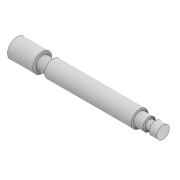
# Autodesk Inventor part: fifth
Saved by Autodesk Inventor 2020 (Build 240168000, 168)
## iProperties
Created: 2021-12-09
Part Number: fifth
Material: Generic
Document SubType Name: Modeling
Designer: NIKHIL VINOD
Density: 1 g/cm^3
Appearance: Default
Author: NIKHIL VINOD
Autodesk Inventor part; units mm, degrees
ref_plane "YZ Plane" through (0, 0, 0) normal (1, 0, 0) x (0, 1, 0)
ref_plane "XZ Plane" through (0, 0, 0) normal (0, 1, 0) x (-1, 0, 0)
ref_plane "XY Plane" through (0, 0, 0) normal (0, 0, 1) x (1, 0, 0)
sketch "Sketch1" plane through (0, 0, 0) normal (0, 0, 1) x (1, 0, 0)
  line L0 (-76.2253, 0) -> (-52.2253, 0)
  line L1 (-52.2253, 6) -> (-52.2253, 9)
  line L2 (-52.2253, 9) -> (-76.2253, 9)
  line L3 (-76.2253, 9) -> (-76.2253, 0)
  line L4 (-52.2253, 0) -> (-42.2253, 0)
  line L5 (-42.2253, 6) -> (-52.2253, 6)
  line L6 (-42.2253, 0) -> (39.7747, 0)
  line L7 (39.7747, 6) -> (39.7747, 8)
  line L8 (39.7747, 8) -> (-42.2253, 8)
  line L9 (-42.2253, 8) -> (-42.2253, 6)
  line L10 (39.7747, 0) -> (48.7747, 0)
  line L11 (48.7747, 4) -> (48.7747, 6)
  line L12 (48.7747, 6) -> (39.7747, 6)
  line L13 (48.7747, 0) -> (54.7747, 0)
  line L14 (54.7747, 4) -> (48.7747, 4)
  line L15 (54.7747, 0) -> (61.7747, 0)
  line L16 (61.7747, 0) -> (61.7747, 6)
  line L17 (61.7747, 6) -> (54.7747, 6)
  line L18 (54.7747, 6) -> (54.7747, 4)
  point P0 (0, 0)
  dimension "d0" = 24
  dimension "d1" = 9
  dimension "d2" = 10
  dimension "d3" = 6
  dimension "d4" = 82
  dimension "d5" = 8
  dimension "d6" = 9
  dimension "d7" = 6
  dimension "d8" = 4
  dimension "d9" = 7
  dimension "d10" = 6
  constraints: 38 end point, 9 parallel, 6 horizontal, 4 perpendicular
  measures "d0" distance of L2.end L1.end
  measures "d1" distance of L1.end L0.end
  measures "d2" distance of L1.start L5.start
  measures "d3" distance of L5.start L4.end
  measures "d4" distance of L8.end L7.end
  measures "d5" distance of L7.end L6.end
  measures "d6" distance of L7.start L11.end
  measures "d7" distance of L14.start L11.start
  measures "d8" distance of L14.start L13.end
  measures "d9" distance of L17.end L16.end
  measures "d10" distance of L16.end L15.end
revolve "Revolution1" add sketch "Sketch1" angle 360 about axis through (-52.2253, 0, 0) along (1, 0, 0)
body "Solid1"
